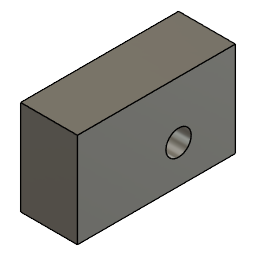
replay (Autodesk Fusion 360 design; units mm, degrees)
Autodesk Fusion 360 part; units mm, degrees
sketch "草图1" plane through (0, 0, 0) normal (1, 0, 0) x (0, 0, -1)
  line L0 (50, 30) -> (0, 30)
  line L1 (0, 30) -> (0, 0)
  line L2 (0, 0) -> (50, 0)
  line L3 (50, 0) -> (50, 30)
extrude "拉伸1" add sketch "草图1" along normal blind 18
sketch "草图2" plane through (18, 0, 0) normal (1, 0, 0) x (0, 0, -1)
  line L0 (50, 0) -> (50, 30)
  line L1 (50, 30) -> (0, 30)
  line L2 (0, 30) -> (0, 0)
  line L3 (0, 0) -> (50, 0)
  circle A0 centre (32, 12) radius 4
extrude "拉伸2" cut sketch "草图2" against normal through all contours A0
